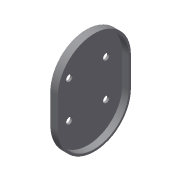
# Autodesk Inventor part: Anténní držák
Saved by Autodesk Inventor 2015 (Build 190159000, 159)
## iProperties
Created: 2015-01-15
Part Number: Anténní držák
Material: Všeobecné
Document SubType Name: Modeling
Designer: Michal
Density: 1 g/cm^3
Appearance: Výchozí
Author: Michal
Autodesk Inventor part; units mm, degrees
ref_plane "YZ Plane" through (0, 0, 0) normal (1, 0, 0) x (0, 1, 0)
ref_plane "XZ Plane" through (0, 0, 0) normal (0, 1, 0) x (-1, 0, 0)
ref_plane "XY Plane" through (0, 0, 0) normal (0, 0, 1) x (1, 0, 0)
sketch "Náčrt1" plane through (0, 0, 0) normal (1, 0, 0) x (0, 1, 0)
  line L0 (50, 70) -> (-50, 70)
  line L1 (-50, 70) -> (-50, -70)
  line L2 (-50, -70) -> (50, -70)
  line L3 (50, -20) -> (50, 70)
  arc A0 (50, 20) -> (-50, 20) centre (0, 20) ccw
  arc A1 (-50, -20) -> (50, -20) centre (0, -20) ccw
  point P0 (0, 0)
  dimension "d0" = 100
  dimension "d1" = 140
  dimension "d2" = 50
  dimension "d3" = 70
  dimension "d4" = 100
  dimension "d8" = 100
  constraints: 8 end point, 4 point on circle, 3 point on line, 3 tangent, 2 centre point, 2 parallel, 1 horizontal, 1 perpendicular
  measures "d0" distance of L2.end L1.end
  measures "d1" distance of L1.end L0.end
  measures "d2" distance from line of L3 point (0, 0)
  measures "d3" distance from line of L0 point (0, 0)
  measures "d4" diameter of A0
  measures "d8" diameter of A1
extrude "Vysunutí2" add sketch "Náčrt1" along normal blind 12 contours A0 L3 A1 L1
sketch "Náčrt2" plane through (12, 0, 0) normal (1, 0, 0) x (0, 0, -1)
  arc A0 (-20, 50) -> (-20, -50) centre (-20, 0) ccw projected
  line L0 (-20, -50) -> (20, -50) projected
  arc A1 (20, -50) -> (20, 50) centre (20, 0) ccw projected
  line L1 (20, 50) -> (-20, 50) projected
  arc A2 (-20, 47) -> (-20, -47) centre (-20, 0) ccw
  line L2 (-20, -47) -> (20, -47)
  arc A3 (20, -47) -> (20, 47) centre (20, 0) ccw
  line L3 (20, 47) -> (-20, 47)
  point P0 (0, 0)
  dimension "d11" = 3
  constraints: 4 end point, 4 point on circle, 2 centre point, 3 other
  measures "d11" distance between parallel lines of L1 L3
extrude "Vysunutí3" cut sketch "Náčrt2" against normal blind 9 contours L3 A3 L2 A2
sketch "Náčrt4" plane through (0, 0, 0) normal (-1, 0, 0) x (0, 0, 1)
  circle A0 centre (25.25, -25.25) radius 4.25
  arc A1 (20, -50) -> (20, 50) centre (20, 0) ccw projected
  line L0 (-20, 50) -> (20, 50) projected
  arc A2 (-20, 50) -> (-20, -50) centre (-20, 0) ccw projected
  line L1 (20, -50) -> (-20, -50) projected
  arc A3 (20, -50) -> (20, 50) centre (20, 0) ccw projected
  circle A4 centre (25.25, 25.25) radius 4.25
  circle A5 centre (-25.25, 25.25) radius 4.25
  circle A6 centre (-25.25, -25.25) radius 4.25
  point P0 (0, 0)
  point P1 (70, 0)
  dimension "d25" = 8.5
  dimension "d26" = 24.75
  dimension "d27" = 44.75
  dimension "d32" = 360
  constraints: 4 centre point, 2 point on circle, 9 other
  measures "d25" diameter of A0
  measures "d26" distance from line of L1 A0.centre
  measures "d27" horizontal distance of point (70, 0) A0.centre
extrude "Vysunutí5" cut sketch "Náčrt4" against normal through all contours A0 | A4 | A5 | A6
fillet "Zaoblení2" radius 3 4 edges at (0, -50, 0) (0, 0, -70) (0, 50, 0) (0, 0, 70)
